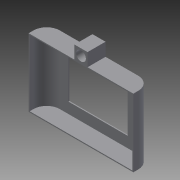
# Autodesk Inventor part: Back
Saved by Autodesk Inventor 2015 SP1 (Build 190203100, 203)
## iProperties
Created: 2015-05-03
Part Number: Back
Material: Generic
Document SubType Name: Modeling
Designer: Brandon
Density: 1 g/cm^3
Appearance: Default
Author: Brandon
Autodesk Inventor part; units mm, degrees
ref_plane "YZ Plane" through (0, 0, 0) normal (1, 0, 0) x (0, 1, 0)
ref_plane "XZ Plane" through (0, 0, 0) normal (0, 1, 0) x (-1, 0, 0)
ref_plane "XY Plane" through (0, 0, 0) normal (0, 0, 1) x (1, 0, 0)
sketch "Sketch1" plane through (0, 0, 0) normal (0, 0, 1) x (1, 0, 0)
  line L0 (28.8, -21.6) -> (-28.8, -21.6)
  line L1 (-28.8, -21.6) -> (-28.8, 21.6)
  line L2 (-28.8, 21.6) -> (28.8, 21.6)
  line L3 (28.8, 21.6) -> (28.8, -21.6)
  line L4 (28.8, -21.6) -> (-28.8, 21.6) construction
  line L5 (-28.8, -21.6) -> (28.8, 21.6) construction
  line L6 (-34.3, -26.7) -> (34.3, -26.7)
  line L7 (34.3, -26.7) -> (34.3, 26.7)
  line L8 (34.3, 26.7) -> (-34.3, 26.7)
  line L9 (-34.3, 26.7) -> (-34.3, -26.7)
  line L10 (-34.3, -26.7) -> (34.3, 26.7) construction
  line L11 (34.3, -26.7) -> (-34.3, 26.7) construction
  line L12 (-40.65, 33.05) -> (40.65, 33.05)
  line L13 (40.65, 33.05) -> (40.65, -33.05)
  line L14 (40.65, -33.05) -> (-40.65, -33.05)
  line L15 (-40.65, -33.05) -> (-40.65, 33.05)
  line L16 (-50.8, -33.05) -> (50.8, -33.05)
  line L17 (50.8, -33.05) -> (50.8, 33.05)
  line L18 (50.8, 33.05) -> (-50.8, 33.05)
  line L19 (-50.8, 33.05) -> (-50.8, -33.05)
  line L20 (-50.8, -33.05) -> (50.8, 33.05) construction
  line L21 (50.8, -33.05) -> (-50.8, 33.05) construction
  point P0 (0, 0)
  dimension "d0" = 43.2
  dimension "d1" = 57.6
  dimension "d2" = 68.6
  dimension "d3" = 53.4
  dimension "d4" = 6.35
  dimension "d7" = 101.6
  dimension "d8" = 66.1
  constraints: 44 end point, 8 parallel, 6 midpoint, 4 perpendicular, 3 horizontal, 3 other
  measures "d0" distance of L2.end L0.start
  measures "d1" distance of L1.end L2.end
  measures "d2" distance of L7.end L8.end
  measures "d3" distance of L6.end L7.end
  measures "d4" distance between parallel lines of L8 L12
  measures "d7" distance of L17.end L18.end
  measures "d8" distance of L16.end L17.end
extrude "Extrusion1" add sketch "Sketch1" along normal blind 17.4625 contours L9 L8 L7 L6 | L12 L13 L14 L15 | L15 L16 L19 L18 | L18 L17 L16 L13
shell "Shell1" thickness 1 removed faces 5 at (-43.4667, 7.2, 17.4625) at (-28.8, -7.2, 5.8208) at (-9.6, 21.6, 5.8208) at (28.8, 7.2, 5.8208) at (9.6, -21.6, 5.8208)
fillet "Fillet1" radius 12.7 2 edges at (-50.8, 0, 0) (50.8, 0, 0)
sketch "Sketch2" plane through (-50.8, 33.05, 17.4625) normal (0, 1, 0) x (1, 0, 0)
  arc A0 (101.6, 4.7625) -> (88.9, 17.4625) centre (88.9, 4.7625) ccw projected
  line L0 (88.9, 17.4625) -> (12.7, 17.4625) projected
  arc A1 (12.7, 17.4625) -> (0, 4.7625) centre (12.7, 4.7625) ccw projected
  line L1 (0, 4.7625) -> (0, 0) projected
  line L2 (101.6, 0) -> (0, 0) projected
  line L3 (101.6, 4.7625) -> (101.6, 0) projected
  line L4 (101.6, 0) -> (0, 0) construction
  line L5 (50.8, 0) -> (50.8, 17.4625) construction
  line L6 (57.15, 17.4625) -> (44.45, 17.4625)
  line L7 (44.45, 17.4625) -> (44.45, 0)
  line L8 (44.45, 0) -> (57.15, 0)
  line L9 (57.15, 0) -> (57.15, 17.4625)
  dimension "d11" = 12.7
  constraints: 10 end point, 2 parallel, 1 collinear, 1 horizontal, 1 midpoint, 1 perpendicular, 1 point on line, 1 vertical, 1 other
  measures "d11" distance of L7.end L8.end
extrude "Extrusion2" add sketch "Sketch2" along normal blind 12.7 contours L9 L2 L7 L0
sketch "Sketch3" plane through (0, 0, 0) normal (0, 0, -1) x (-1, 0, 0)
  line L0 (-38.1, -33.05) -> (-38.1, 33.05) projected
  line L1 (38.1, -33.05) -> (-38.1, -33.05) projected
  line L2 (38.1, 33.05) -> (38.1, -33.05) projected
  line L3 (6.35, 33.05) -> (38.1, 33.05) projected
  line L4 (6.35, 33.05) -> (6.35, 45.75) projected
  line L5 (-6.35, 45.75) -> (6.35, 45.75) projected
  line L6 (-6.35, 33.05) -> (-6.35, 45.75) projected
  line L7 (-38.1, 33.05) -> (-6.35, 33.05) projected
  line L8 (28.8, 21.6) -> (28.8, -21.6) projected
  line L9 (28.8, -21.6) -> (-28.8, -21.6) projected
  line L10 (-28.8, -21.6) -> (-28.8, 21.6) projected
  line L11 (-28.8, 21.6) -> (28.8, 21.6) projected
  line L12 (-6.35, 45.75) -> (6.35, 33.05) construction
  line L13 (6.35, 33.05) -> (6.35, 45.75) construction
  line L14 (6.35, 45.75) -> (-6.35, 33.05) construction
  point P0 (0, 0)
  point P1 (0, 39.4)
  constraints: 6 end point, 1 collinear, 1 midpoint, 1 perpendicular
hole "Hole1" at (0, 39.4, 0) direction (0, 0, 1) diameter 9.525 end through all
fillet "Fillet2" radius 12.7 2 edges at (-49.8, 0, 1) (49.8, 0, 1)
equation "\"d8\" = 2 * d4 + d3"
body "Solid1"
